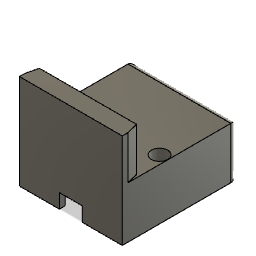
_motor mount.4d701924-e459-45fc-a762-8e1285cabc4e (Autodesk Fusion 360 design; units mm, degrees)
Autodesk Fusion 360 part; units mm, degrees
sketch "reference" plane through (0, 0, 0) normal (0, 1, 0) x (1, 0, 0)
  line L0 (26.708, 42.6236) -> (27.1586, 42.6236)
  line L1 (-27.225, -55.0823) -> (17.225, -55.0823)
  line L2 (17.225, -55.0823) -> (17.225, -42.3823)
  line L3 (17.225, -42.3823) -> (-27.225, -42.3823)
  line L4 (-27.225, -42.3823) -> (-27.225, -55.0823)
  circle A0 centre (0, 0) radius 65
  line L5 (-27.225, 55.0823) -> (17.225, 55.0823)
  line L6 (17.225, 55.0823) -> (17.225, 42.3823)
  line L7 (17.225, 42.3823) -> (-27.225, 42.3823)
  line L8 (-27.225, 55.0823) -> (-27.225, 42.3823)
  circle A1 centre (0, 0) radius 67.15
  circle A2 centre (68.0978, 18.2467) radius 3
  circle A3 centre (68.0978, 18.2467) radius 1.425
  line L9 (0, 0) -> (82, 0) construction
  line L10 (0, 0) -> (-41, 71.0141) construction
  line L11 (0, 0) -> (-41, -71.0141) construction
  line L12 (87.4769, -0.0257) -> (79.614, 0.0081)
  line L13 (-39.814, 68.9437) -> (-43.7162, 75.77)
  line L14 (-39.8, -68.9518) -> (-43.7607, -75.7444)
  line L15 (0, 0) -> (70.5, 0) construction
  arc A4 (79.614, 0.0081) -> (74.6944, -3.9877) centre (79.5926, -4.9919) ccw
  arc A5 (-39.814, 68.9437) -> (-33.8938, 66.6811) centre (-35.4732, 71.4251) ccw
  arc A6 (-39.8, -68.9518) -> (-40.8007, -62.6934) centre (-44.1194, -66.4332) ccw
  spline S0 degree 5 poles (-33.8938, 66.6811) (-33.483, 66.8179) (-33.0729, 66.9532) (-32.6634, 67.087) (-32.2547, 67.2193) (-31.8466, 67.3502) knots 0.021144 0.021144 0.021144 0.021144 0.021144 0.021144 0.032444 0.032444 0.032444 0.032444 0.032444 0.032444
  line L16 (-32.0549, 67.2834) -> (-31.6382, 67.417)
  spline S1 degree 5 poles (5.0849, 74.3263) (6.6179, 74.3731) (11.2429, 74.4207) (18.7539, 74.0099) (28.746, 72.2391) (40.5731, 67.6689) (52.3904, 59.5578) (62.916, 48.5693) (72.252, 34.9305) (78.8493, 22.0782) (83.3385, 11.4171) (86.1309, 3.8631) (87.4769, -0.0257) knots 0.251095 0.251095 0.251095 0.251095 0.251095 0.251095 0.3 0.4 0.5 0.6 0.7 0.8 0.9 1 1 1 1 1 1
  line L17 (-9.3123, 73.8863) -> (19.482, 74.7663)
  spline S2 degree 5 poles (-40.8007, -62.6934) (-41.1245, -62.4061) (-41.4467, -62.1186) (-41.7673, -61.8309) (-42.0863, -61.543) (-42.4037, -61.255) knots 0.021144 0.021144 0.021144 0.021144 0.021144 0.021144 0.032444 0.032444 0.032444 0.032444 0.032444 0.032444
  line L18 (-42.2416, -61.4021) -> (-42.5658, -61.1079)
  spline S3 degree 5 poles (-66.9109, -32.7595) (-67.718, -31.4553) (-70.0717, -27.4737) (-73.4714, -20.7636) (-76.9339, -11.2248) (-78.8895, 1.3029) (-77.7737, 15.5925) (-73.5202, 30.2022) (-66.3767, 45.1068) (-58.5449, 57.2464) (-51.5568, 66.4647) (-46.4109, 72.66) (-43.7162, 75.77) knots 0.251095 0.251095 0.251095 0.251095 0.251095 0.251095 0.3 0.4 0.5 0.6 0.7 0.8 0.9 1 1 1 1 1 1
  line L19 (-59.9171, -44.0611) -> (-73.9047, -21.4578)
  arc A7 (-66.9109, -32.7595) -> (-37.25, -64.5189) centre (0, 0) ccw
  spline S4 degree 5 poles (74.6944, -3.9877) (74.6075, -4.4118) (74.5196, -4.8346) (74.4308, -5.2561) (74.341, -5.6763) (74.2503, -6.0951) knots 0.021144 0.021144 0.021144 0.021144 0.021144 0.021144 0.032444 0.032444 0.032444 0.032444 0.032444 0.032444
  line L20 (74.2965, -5.8814) -> (74.204, -6.3089)
  spline S5 degree 5 poles (61.826, -41.5668) (61.1001, -42.9178) (58.8287, -46.947) (54.7175, -53.2463) (48.1879, -61.0143) (38.3164, -68.9717) (25.3834, -75.1503) (10.6042, -78.7715) (-5.8753, -80.0373) (-20.3044, -79.3246) (-31.7817, -77.8819) (-39.7199, -76.523) (-43.7607, -75.7444) knots 0.251095 0.251095 0.251095 0.251095 0.251095 0.251095 0.3 0.4 0.5 0.6 0.7 0.8 0.9 1 1 1 1 1 1
  line L21 (68.2252, -29.657) -> (55.4268, -53.4766)
  arc A8 (61.826, -41.5668) -> (74.5, 0) centre (0, 0) ccw
  arc A9 (5.0849, 74.3263) -> (-37.25, 64.5189) centre (0, 0) ccw
  circle A10 centre (18.2467, 68.0978) radius 3
  circle A11 centre (18.2467, 68.0978) radius 1.425
  circle A12 centre (-49.851, 49.851) radius 3
  circle A13 centre (-49.851, 49.851) radius 1.425
  circle A14 centre (-68.0978, -18.2467) radius 3
  circle A15 centre (-68.0978, -18.2467) radius 1.425
  circle A16 centre (-18.2467, -68.0978) radius 3
  circle A17 centre (-18.2467, -68.0978) radius 1.425
  circle A18 centre (49.851, -49.851) radius 3
  circle A19 centre (49.851, -49.851) radius 1.425
  line L22 (0, 0) -> (55.15, 0) construction
  line L23 (0, 0) -> (55.15, 0) construction
  circle A20 centre (42.2474, -35.4497) radius 12
  circle A21 centre (42.2474, 35.4497) radius 12
  line L24 (0, 0) -> (55.15, 0) construction
  line L25 (0, 0) -> (55.15, 0) construction
  circle A22 centre (-42.2474, 35.4497) radius 12
  circle A23 centre (-42.2474, -35.4497) radius 12
  circle A24 centre (0, 0) radius 62.5
  line L26 (-5, -42.3823) -> (-5, 42.3823)
  point P0 (39, 67.55)
  point P1 (-78, 0)
  point P2 (39, -67.55)
  dimension "d9" = 12.7
  dimension "d10" = 44.45
  dimension "d53" = 12.7
  dimension "d54" = 44.45
  dimension "d63" = 130
  dimension "d76" = 134.3
  dimension "d123" = 78
  dimension "d127" = 5
  dimension "d128" = 5
  dimension "d129" = 5
  dimension "d132" = 149
  dimension "d136" = 360
  dimension "d204" = 55.15
  dimension "d206" = 55.15
  dimension "d207" = 24
  dimension "d208" = 24
  dimension "d210" = 55.15
  dimension "d212" = 55.15
  dimension "d213" = 24
  dimension "d214" = 24
  dimension "d227" = 125
  dimension "d232" = 84.7646
  constraint perpendicular L1 L2
  constraint perpendicular L2 L3
  constraint coincident A0.centre A1.centre
  constraint perpendicular L5 L6
  constraint perpendicular L6 L7
  constraint horizontal L9
  constraint horizontal L15
  constraint tangent A4 S4
  constraint tangent L12 A4
  constraint tangent A5 S0
  constraint tangent L13 A5
  constraint tangent A6 S2
  constraint tangent L14 A6
  constraint coincident S0.end A7
  constraint midpoint S0.end L16
  constraint coincident S1.start A7
  constraint midpoint S1.start L17
  constraint coincident L10 A9.end
  constraint coincident S2.end A7
  constraint midpoint S2.end L18
  constraint midpoint S3.start L19
  constraint coincident L11 A7.end
  constraint concentric A7 A8
  constraint coincident S4.end A8
  constraint midpoint S4.end L20
  constraint midpoint S5.start L21
  constraint coincident L9 A8.end
  constraint concentric A8 A9
  constraint horizontal L22
  constraint horizontal L23
  constraint horizontal L24
  constraint horizontal L25
  constraint midpoint L3 L26.start
  constraint midpoint L7 L26.end
  constraint perpendicular L7 L26
  measures "d9" distance of L1.end L2.end
  measures "d10" distance of L2.end L3.end
  measures "d53" distance of L5.end L6.end
  measures "d54" distance of L6.end L7.end
  measures "d63" diameter of A0
  measures "d76" diameter of A1
  measures "d123" distance of A0.centre P0
  measures "d127" radius of A4
  measures "d128" radius of A5
  measures "d129" radius of A6
  measures "d132" diameter of A7
  measures "d204" distance of A0.centre A20.centre
  measures "d206" distance of A0.centre A21.centre
  measures "d207" diameter of A20
  measures "d208" diameter of A21
  measures "d210" distance of A0.centre A23.centre
  measures "d212" distance of A0.centre A22.centre
  measures "d213" diameter of A22
  measures "d214" diameter of A23
  measures "d227" diameter of A24
  measures "d232" distance of L26.start L26.end
sketch "Sketch6" plane through (0, 0, 0) normal (0, 1, 0) x (1, 0, 0)
  line L0 (7.0001, -41.0033) -> (-11, -41.0033)
  line L1 (-2, -39.9998) -> (-7, -39.9998)
  line L2 (-2, -39.9998) -> (3, -39.9998)
  line L3 (3, -39.9998) -> (3, -20.9998)
  line L4 (-7, -39.9998) -> (-7, -20.9998)
  line L5 (-11, -20.9998) -> (7.0001, -20.9998)
  line L6 (0, -40.9998) -> (0, -39.9998)
  line L7 (-4, -40.9998) -> (-4, -39.9998)
  circle A0 centre (5.5279, -32.9998) radius 1.425
  circle A1 centre (-9.5, -33) radius 1.425
  line L8 (-11, -20.9998) -> (-11, -41.0033)
  line L9 (-4, -41.0033) -> (-4, -39.9998)
  line L10 (0, -41.0033) -> (0, -39.9998)
  line L11 (7.0001, -38) -> (-11, -38)
  line L12 (7.0001, -20.9998) -> (7.0001, -41.0033)
  point P0 (-9.5, -33)
  point P1 (5.5279, -32.9998)
  dimension "d334" = 19
  dimension "d549" = 2.85
  dimension "d552" = 2.85
  constraint horizontal L0
  constraint perpendicular L2 L3
  constraint perpendicular L1 L4
  constraint perpendicular L4 L5
  constraint coincident L4.end L5
  constraint coincident L3.end L5
  constraint perpendicular L0 L8
  constraint perpendicular L0 L9
  constraint perpendicular L2 L10
  constraint coincident L0 L9.start
  constraint coincident L7.start L9
  constraint coincident L0 L10.start
  constraint coincident L6.start L10
  constraint coincident L8 L11.end
  constraint horizontal L11
  measures "d334" distance of L2.end L3.end
  measures "d549" diameter of A0
  measures "d552" diameter of A1
extrude "Extrude186" add sketch "Sketch6" along normal blind 9 from surface at -9.1 contours L0 L2 L3 L6 L10 L11 L12 | L3 L5 L11 L12 | L0 L1 L4 L7 L8 L9 L11 | L4 L5 L8 L11 makes body 1 at (-11, -3.1, 27.6676) makes body 2 at (7.0001, -3.1, 27.6676)
extrude "Extrude187" add sketch "Sketch6" against normal blind 6.6 contours L0 L1 L2 L6 L7 L9 L10 bodies 1 2
extrude "Extrude188" add sketch "Sketch6" against normal blind 3 from surface at -0.1 separate body contours L3 L4 L5 L11 | L1 L2 L3 L4 L11 makes body 3
extrude "Extrude189" add sketch "Sketch6" along normal blind 8.5 from surface at -1 contours L0 L2 L3 L6 L10 L11 L12 | L0 L1 L2 L6 L7 L9 L10 | L0 L1 L4 L7 L8 L9 L11 | L1 L2 L3 L4 L11 bodies 1 3
extrude "Extrude190" add sketch "Sketch6" against normal blind 9.1 contours L0 L2 L3 L6 L10 L11 L12 | L0 L1 L4 L7 L8 L9 L11 bodies 1
fillet "Fillet203" radius 1 4 edges at (7.0001, -4.6, 20.9998) (5.0001, -0.1, 20.9998) (-9, -0.1, 20.9998) (-11, -4.6, 20.9998) on bodies 1
chamfer "Chamfer12" distance 0.5 distance2 2 1 edges at (-11, 3.7, 38) measured on face at (-4.9999, 4.9667, 38) on bodies 1
chamfer "Chamfer13" distance 2 distance2 0.5 1 edges at (7.0001, 3.7, 38) measured on face at (7.0001, -6.1, 33.6677) on bodies 1
